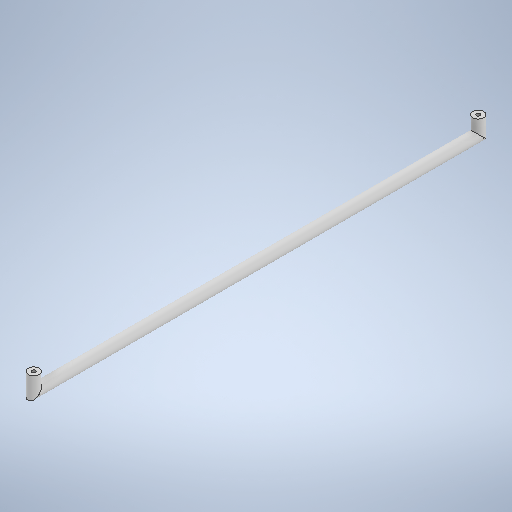
# Autodesk Inventor part: Solar_Panel_Bar
Saved by Autodesk Inventor 2025 (Build 290162010, 162A)
## iProperties
Created: 2024-07-15
Part Number: Solar_Panel_Bar
Material: Generic
Document SubType Name: Modeling
Designer: vncnt
Density: 1 g/cm^3
Appearance: Default
Author: vncnt
Autodesk Inventor part; units mm, degrees
ref_plane "YZ Plane" through (0, 0, 0) normal (1, 0, 0) x (0, 1, 0)
ref_plane "XZ Plane" through (0, 0, 0) normal (0, 1, 0) x (-1, 0, 0)
ref_plane "XY Plane" through (0, 0, 0) normal (0, 0, 1) x (1, 0, 0)
sketch "Sketch1" plane through (0, 0, 0) normal (0, 0, 1) x (1, 0, 0)
  circle A0 centre (0, 0) radius 3.175
  dimension "d0" = 6.35
  constraints: 1 centre point, 1 coincident
  measures "d0" diameter of A0
extrude "Extrusion1" add sketch "Sketch1" along normal mid plane 259
sketch "Sketch2" plane through (0, 0, 0) normal (0, 1, 0) x (-1, 0, 0)
  circle A0 centre (0, 129.875) radius 3.175
  circle A1 centre (0, -129.875) radius 3.175
  line L0 (-3.175, -129.5) -> (-3.175, 129.5) projected
  line L1 (-3.175, 0) -> (16.7407, 0)
  point P0 (3.175, -105.625)
  dimension "d4" = 259.75
  dimension "d5" = 129.875
  dimension "d6" = 6.35
  dimension "d7" = 6.35
  constraints: 2 centre point, 2 end point, 1 horizontal, 1 midpoint
  measures "d4" distance of A0.centre A1.centre
  measures "d5" distance from line of L1 A0.centre
  measures "d6" diameter of A0
  measures "d7" diameter of A1
extrude "Extrusion2" add sketch "Sketch2" along normal blind 10 and the other way blind 3.175
sketch "Sketch3" plane through (0, 10, 129.875) normal (0, 1, 0) x (1, 0, 0)
  circle A0 centre (0, 0) radius 3.175 projected
  circle A1 centre (0, 259.75) radius 3.175 projected
  point P0 (0, 129.875)
  constraints: 2 coincident
hole "Hole1" at (0, 10, 129.875) at (0, 10, -129.875) direction (0, -1, 0) diameter 2.1565 end through all thread size "4-40 UNC" class "2B" standard "ANSI Unified Screw Threads"
sketch "Sketch6" plane through (0, 0, 0) normal (0, 0, 1) x (1, 0, 0)
  arc A0 (-3.1528, -0.375) -> (0, -3.175) centre (0, 0) ccw projected
  circle A1 centre (0, 0) radius 3.175
  line L0 (-3.175, -3.175) -> (3.175, -3.175) projected
  line L1 (-3.175, -3.175) -> (3.175, -3.175)
  line L2 (3.175, -3.175) -> (3.175, 0)
  line L3 (3.175, 0) -> (-3.175, 0)
  line L4 (-3.175, 0) -> (-3.175, -3.175)
  point P0 (0, -3.175)
  point P1 (0, -3.175)
  point P2 (-3.175, 0)
  constraints: 8 end point, 2 parallel, 2 point on circle, 1 centre point, 1 coincident, 1 horizontal, 1 perpendicular
extrude "Extrusion5" cut sketch "Sketch6" along normal through all both and the other way through all contours A1 L2 L0
body "Solid1"
